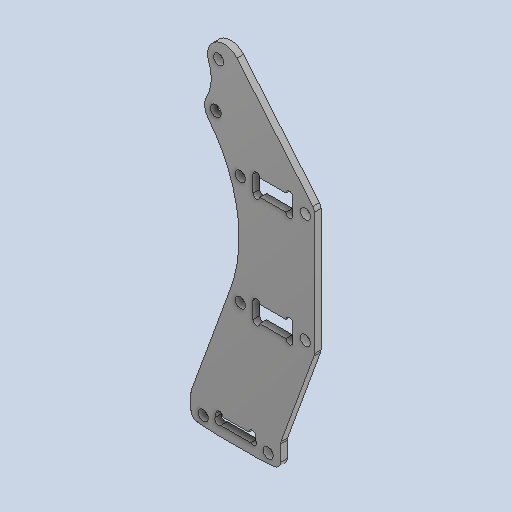
# Autodesk Inventor part: Head_side_frame
Saved by Autodesk Inventor 2022.4 (Build 264492000, 492)
## iProperties
Created: 2021-09-02
Part Number: Head_side_frame
Material: GFRP
Document SubType Name: Modeling
Designer: Masato
Density: 1.75 g/cm^3
Appearance: 滑らか - 標準の灰色
Mass: 7.67841 g
Surface Area: 52.6786 cm^2
Volume: 4.38766 cm^3
Description: GFRP T2
Author: Masato Kubotera
Autodesk Inventor part; units mm, degrees
ref_plane "YZ Plane" through (0, 0, 0) normal (1, 0, 0) x (0, 1, 0)
ref_plane "XZ Plane" through (0, 0, 0) normal (0, 1, 0) x (-1, 0, 0)
ref_plane "XY Plane" through (0, 0, 0) normal (0, 0, 1) x (1, 0, 0)
sketch "スケッチ1" plane through (0, 0, 0) normal (0, 0, 1) x (1, 0, 0)
  line L0 (0, 0) -> (27, 0) construction
  line L1 (27, 0) -> (27, 5) construction
  line L2 (27, 5) -> (0, 5) construction
  line L3 (0, 5) -> (0, 0) construction
  line L4 (0, 2.5) -> (27, 2.5) construction
  line L5 (13.5, 5) -> (13.5, 0) construction
  circle A0 centre (3.7, 2.5) radius 1.55
  line L6 (7.5, 5) -> (7.5, 0) construction
  circle A1 centre (23.3, 2.5) radius 1.55
  line L7 (19.5, 5) -> (19.5, 0) construction
  line L8 (7.49, 5.01) -> (9.59, 5.01) construction
  line L9 (19.51, 5.01) -> (19.51, 2.49)
  line L10 (19.51, 2.49) -> (7.49, 2.49)
  line L11 (7.49, 2.49) -> (7.49, 5.01)
  line L12 (7.49, 5.01) -> (19.51, 2.49) construction
  line L13 (19.51, 5.01) -> (7.49, 2.49) construction
  arc A2 (9.59, 5.01) -> (7.49, 5.01) centre (8.54, 5.01) ccw
  arc A3 (19.51, 5.01) -> (17.41, 5.01) centre (18.46, 5.01) ccw
  line L14 (9.59, 5.01) -> (17.41, 5.01)
  line L15 (9.59, 2.49) -> (7.49, 2.49)
  line L16 (17.41, 5.01) -> (19.51, 5.01) construction
  line L17 (27, 7) -> (0, 7) construction
  line L18 (0, 0) -> (0, 7)
  line L19 (12.1912, 35) -> (37.1912, 35) construction
  line L20 (37.1912, 35) -> (37.1912, 40) construction
  line L21 (37.1912, 40) -> (12.1912, 40) construction
  line L22 (12.1912, 40) -> (12.1912, 35) construction
  line L23 (12.1912, 37.5) -> (37.1912, 37.5) construction
  line L24 (24.6912, 40) -> (24.6912, 35) construction
  circle A4 centre (14.8912, 37.5) radius 1.55
  line L25 (18.6912, 40) -> (18.6912, 35) construction
  line L26 (30.6912, 40) -> (30.6912, 35) construction
  circle A5 centre (34.4912, 37.5) radius 1.55
  line L27 (18.6812, 40.01) -> (20.7812, 40.01) construction
  line L28 (30.7012, 40.01) -> (30.7012, 34.99)
  line L29 (30.7012, 34.99) -> (28.6012, 34.99) construction
  line L30 (18.6812, 34.99) -> (18.6812, 40.01)
  line L31 (18.6812, 40.01) -> (30.7012, 34.99) construction
  line L32 (30.7012, 40.01) -> (18.6812, 34.99) construction
  arc A6 (20.7812, 40.01) -> (18.6812, 40.01) centre (19.7312, 40.01) ccw
  arc A7 (18.6812, 34.99) -> (20.7812, 34.99) centre (19.7312, 34.99) ccw
  arc A8 (30.7012, 40.01) -> (28.6012, 40.01) centre (29.6512, 40.01) ccw
  arc A9 (28.6012, 34.99) -> (30.7012, 34.99) centre (29.6512, 34.99) ccw
  line L33 (20.7812, 40.01) -> (28.6012, 40.01)
  line L34 (20.7812, 34.99) -> (18.6812, 34.99) construction
  line L35 (28.6012, 40.01) -> (30.7012, 40.01) construction
  line L36 (28.6012, 34.99) -> (20.7812, 34.99)
  line L37 (12.1912, 73) -> (12.1912, 68) construction
  circle A10 centre (14.8912, 70.5) radius 1.55
  line L38 (37.1912, 68) -> (37.1912, 73) construction
  line L39 (30.6912, 73) -> (30.6912, 68) construction
  circle A11 centre (34.4912, 70.5) radius 1.55
  line L40 (30.7012, 73.01) -> (30.7012, 67.99)
  line L41 (18.6912, 73) -> (18.6912, 68) construction
  line L42 (12.1912, 68) -> (37.1912, 68) construction
  line L43 (37.1912, 73) -> (12.1912, 73) construction
  line L44 (12.1912, 70.5) -> (37.1912, 70.5) construction
  line L45 (24.6912, 73) -> (24.6912, 68) construction
  line L46 (20.7812, 73.01) -> (28.6012, 73.01)
  line L47 (28.6012, 67.99) -> (20.7812, 67.99)
  line L48 (18.6812, 73.01) -> (30.7012, 67.99) construction
  line L49 (30.7012, 73.01) -> (18.6812, 67.99) construction
  arc A12 (30.7012, 73.01) -> (28.6012, 73.01) centre (29.6512, 73.01) ccw
  line L50 (28.6012, 73.01) -> (30.7012, 73.01) construction
  arc A13 (28.6012, 67.99) -> (30.7012, 67.99) centre (29.6512, 67.99) ccw
  line L51 (30.7012, 67.99) -> (28.6012, 67.99) construction
  line L52 (18.6812, 73.01) -> (20.7812, 73.01) construction
  line L53 (20.7812, 67.99) -> (18.6812, 67.99) construction
  arc A14 (20.7812, 73.01) -> (18.6812, 73.01) centre (19.7312, 73.01) ccw
  arc A15 (18.6812, 67.99) -> (20.7812, 67.99) centre (19.7312, 67.99) ccw
  line L54 (18.6812, 67.99) -> (18.6812, 73.01)
  line L55 (27, 0) -> (27, 6.6473)
  line L56 (37.1912, 35) -> (27.1206, 7.3314)
  line L57 (11.8992, 39.6929) -> (0, 7)
  line L58 (37.1912, 35) -> (37.1912, 73)
  line L59 (6.8054, 101.4338) -> (6.7491, 101.3865)
  arc A16 (4.7394, 86.3065) -> (5.3203, 95.7003) centre (-4.8938, 91.617) ccw
  circle A17 centre (-4.8938, 91.617) radius 14.6063 construction
  line L60 (1.0459, 61.9185) -> (-21.5815, 84.5459) construction
  line L61 (-21.5815, 84.5459) -> (-18.0459, 88.0815) construction
  line L62 (-18.0459, 88.0815) -> (4.5815, 65.4541) construction
  line L63 (4.5815, 65.4541) -> (1.0459, 61.9185) construction
  line L64 (1.0459, 61.9185) -> (-18.0459, 88.0815) construction
  line L65 (-21.5815, 84.5459) -> (4.5815, 65.4541) construction
  line L66 (13.8495, 100.8175) -> (37.1912, 73)
  arc A18 (11.8992, 39.6929) -> (5.2055, 80.7796) centre (-28.1256, 54.2607) ccw
  arc A19 (8.344, 97.7899) -> (6.2953, 101.0057) centre (-4.8938, 91.617) ccw construction
  arc A20 (5.0756, 80.942) -> (7.4988, 83.886) centre (-4.8938, 91.617) ccw construction
  circle A21 centre (8.344, 97.7899) radius 1.55
  circle A22 centre (7.4988, 83.886) radius 1.65
  arc A23 (13.8495, 100.8175) -> (6.8054, 101.4338) centre (10.0193, 97.6035) ccw
  arc A24 (6.7491, 101.3865) -> (5.3203, 95.7003) centre (9.9631, 97.5563) ccw
  arc A25 (4.7394, 86.3065) -> (5.2055, 80.7796) centre (9.1182, 83.8926) ccw
  arc A26 (27.1206, 7.3314) -> (27, 6.6473) centre (29, 6.6473) ccw
  arc A27 (7.49, 3.9749) -> (8.9749, 2.49) centre (8.2325, 3.2325) ccw
  arc A28 (18.0251, 2.49) -> (19.51, 3.9749) centre (18.7675, 3.2325) ccw
  line L67 (0, 0) -> (7.5, -0.5)
  line L68 (7.5, -0.5) -> (19.5, -0.5)
  line L69 (27, 0) -> (19.5, -0.5)
  point P0 (24.6912, 37.5)
  point P1 (24.6912, 70.5)
  point P2 (10.6356, 104.6477)
  point P3 (3.5327, 98.6877)
  point P4 (-8.5, 75)
  point P5 (19.51, 3.9749)
  point P6 (18.0251, 2.49)
  point P7 (5.8711, 81.4297)
  dimension "d0" = 27
  dimension "d1" = 5
  dimension "d2" = 3.1
  dimension "d3" = 12
  dimension "d4" = 19.6
  dimension "d9" = 1.05
  dimension "d10" = 7
  dimension "d11" = 25
  dimension "d12" = 5
  dimension "d13" = 3.1
  dimension "d14" = 12
  dimension "d15" = 19.6
  dimension "d16" = 0.01
  dimension "d17" = 0.01
  dimension "d20" = 1.05
  dimension "d22" = 25
  dimension "d23" = 5
  dimension "d24" = 3.1
  dimension "d25" = 12
  dimension "d26" = 19.6
  dimension "d27" = 0.01
  dimension "d28" = 0.01
  dimension "d29" = 1.05
  dimension "d30" = 70
  dimension "d31" = 66
  dimension "d32" = 33
  dimension "d37" = 5
  dimension "d38" = 75
  dimension "d39" = 135
  dimension "d40" = 8.5
  dimension "d46" = 11.8
  dimension "d47" = 32
  dimension "d48" = 50
  dimension "d49" = 6.8
  dimension "d50" = 11
  dimension "d51" = 29.2126
  dimension "d54" = 15
  dimension "d55" = 15
  dimension "d56" = 3.1
  dimension "d57" = 3.3
  dimension "d60" = 5
  dimension "d61" = 2
  dimension "d62" = 1.05
  dimension "d64" = 2.52
  dimension "d65" = 0.01
  dimension "d66" = 0.01
  dimension "d67" = 0.5
  dimension "d69" = 12
  constraints: 140 end point, 48 point on circle, 36 parallel, 29 centre point, 27 symmetric about line, 23 midpoint, 20 point on line, 18 perpendicular, 14 horizontal, 9 tangent, 4 equal radius, 3 coincident, 1 collinear, 1 line through centre, 1 vertical, 12 other
  measures "d0" distance of L2.end L1.end
  measures "d1" distance of L1.end L0.end
  measures "d2" diameter of A0
  measures "d3" distance of L7.end L6.end
  measures "d4" distance of A1.centre A0.centre
  measures "d9" radius of A2
  measures "d10" distance of L0.start L17.end
  measures "d11" distance of L22.start L20.end
  measures "d12" distance of L20.end L20.start
  measures "d13" diameter of A4
  measures "d14" distance of L26.end L25.end
  measures "d15" distance of A5.centre A4.centre
  measures "d16" horizontal distance of L25.start L31.start
  measures "d17" distance from line of L27 L25.start
  measures "d20" radius of A6
  measures "d22" distance of L43.start L43.end
  measures "d23" distance of L43.start L42.end
  measures "d24" diameter of A10
  measures "d25" distance of L39.end L41.end
  measures "d26" distance of A11.centre A10.centre
  measures "d27" horizontal distance of L41.start L54.end
  measures "d28" distance from line of L52 L41.start
  measures "d29" radius of A14
  measures "d30" angle of L17 L56
  measures "d31" vertical distance of L43.start L17.start
  measures "d32" vertical distance of L17.start L20.end
  measures "d37" distance of L60.end L61.end
  measures "d38" vertical distance of point (-8.5, 75) L0.start
  measures "d39" angle of L60 L3
  measures "d40" horizontal distance of L0.start point (-8.5, 75)
  measures "d46" distance from line of A17.centre L62
  measures "d47" distance of L60.start L60.end
  measures "d48" angle of L0 L66
  measures "d49" distance from line of A16.centre L61
  measures "d50" radius of A16
  measures "d51" diameter of A17
  measures "d56" diameter of A21
  measures "d57" diameter of A22
  measures "d60" radius of A23
  measures "d61" radius of A26
  measures "d62" radius of A27
  measures "d64" distance between parallel lines of L10 L16
  measures "d65" distance between parallel lines of L2 L8
  measures "d66" distance between parallel lines of L11 L6
  measures "d67" distance between parallel lines of L68 L0
  measures "d69" distance of L67.end L68.end
extrude "押し出し1" add sketch "スケッチ1" against normal blind 2
fillet "フィレット1" radius 2 5 edges at (37.1912, 73, -1) (37.1912, 35, -1) (0, 7, -1) (27, 0, -1) (0, 0, -1)
equation "\"d12\" = d1"
equation "\"d13\" = d2"
equation "\"d14\" = d3"
equation "\"d15\" = d4"
equation "\"d16\" = d6"
equation "\"d17\" = d6"
equation "\"d22\" = d11"
equation "\"d23\" = d1"
equation "\"d24\" = d2"
equation "\"d25\" = d3"
equation "\"d26\" = d4"
equation "\"d27\" = d6"
equation "\"d28\" = d6"
equation "\"d32\" = 0.5 * d31"
equation "\"d6\" = 0.01"
